Autodesk Inventor part; units mm, degrees
(part 2 of 3)
  spline S240 degree 2 poles (85.4403, 60.8078) (85.4403, 61.153) (85.7516, 61.6651) (86.3259, 61.9367) (86.6994, 61.9367) knots 0 0 0 1 2 3 3 3
  spline S241 degree 2 poles (86.6994, 61.9367) (87.087, 61.9367) (87.6557, 61.651) (87.9584, 61.1445) (87.9584, 60.8333) knots 0 0 0 1 2 3 3 3
  spline S242 degree 2 poles (87.0389, 60.8276) (87.0389, 61.2718) (86.6994, 61.2718) knots 0 0 0 1 1 1
  spline S243 degree 2 poles (86.6994, 61.2718) (86.3599, 61.2718) (86.3599, 60.8078) knots 0 0 0 1 1 1
  spline S244 degree 2 poles (86.3599, 60.8078) (86.3599, 60.3155) (86.705, 60.3155) knots 0 0 0 1 1 1
  spline S245 degree 2 poles (86.705, 60.3155) (87.0389, 60.3155) (87.0389, 60.8276) knots 0 0 0 1 1 1
  line L291 (89.7098, 59.7044) -> (89.7098, 60.8927)
  spline S246 degree 2 poles (89.7098, 60.8927) (89.7098, 61.0964) (89.5881, 61.2718) (89.4523, 61.2718) knots 0 0 0 1 2 2 2
  spline S247 degree 2 poles (89.4523, 61.2718) (89.3363, 61.2718) (89.2033, 61.0879) (89.2033, 60.9465) knots 0 0 0 1 2 2 2
  line L292 (89.2033, 60.9465) -> (89.2033, 59.7044)
  line L293 (89.2033, 59.7044) -> (88.2979, 59.7044)
  line L294 (88.2979, 59.7044) -> (88.2979, 61.883)
  line L295 (88.2979, 61.883) -> (89.2033, 61.883)
  line L296 (89.2033, 61.883) -> (89.2033, 61.5434)
  line L297 (89.2033, 61.5434) -> (89.2118, 61.5434)
  spline S248 degree 2 poles (89.2118, 61.5434) (89.3193, 61.7302) (89.6871, 61.9367) (89.9022, 61.9367) knots 0 0 0 1 2 2 2
  spline S249 degree 2 poles (89.9022, 61.9367) (90.6151, 61.9367) (90.6151, 61.0342) knots 0 0 0 1 1 1
  line L298 (90.6151, 61.0342) -> (90.6151, 59.7044)
  line L299 (90.6151, 59.7044) -> (89.7098, 59.7044)
  line L300 (91.0254, 59.7044) -> (91.0254, 61.883)
  line L301 (91.0254, 61.883) -> (91.9308, 61.883)
  line L302 (91.9308, 61.883) -> (91.9308, 59.7044)
  line L303 (91.9308, 59.7044) -> (91.0254, 59.7044)
  spline S250 degree 2 poles (91.9845, 62.4715) (91.9845, 62.2791) (91.7044, 62.0414) (91.4781, 62.0414) knots 0 0 0 1 2 2 2
  spline S251 degree 2 poles (91.4781, 62.0414) (91.2574, 62.0414) (90.9745, 62.2875) (90.9745, 62.4715) knots 0 0 0 1 2 2 2
  spline S252 degree 2 poles (90.9745, 62.4715) (90.9745, 62.6582) (91.2489, 62.8902) (91.4781, 62.8902) knots 0 0 0 1 2 2 2
  spline S253 degree 2 poles (91.4781, 62.8902) (91.7044, 62.8902) (91.9845, 62.6582) (91.9845, 62.4715) knots 0 0 0 1 2 2 2
  line L304 (93.7783, 59.7044) -> (93.7783, 60.8927)
  spline S254 degree 2 poles (93.7783, 60.8927) (93.7783, 61.0964) (93.6567, 61.2718) (93.5209, 61.2718) knots 0 0 0 1 2 2 2
  spline S255 degree 2 poles (93.5209, 61.2718) (93.4048, 61.2718) (93.2719, 61.0879) (93.2719, 60.9465) knots 0 0 0 1 2 2 2
  line L305 (93.2719, 60.9465) -> (93.2719, 59.7044)
  line L306 (93.2719, 59.7044) -> (92.3665, 59.7044)
  line L307 (92.3665, 59.7044) -> (92.3665, 61.883)
  line L308 (92.3665, 61.883) -> (93.2719, 61.883)
  line L309 (93.2719, 61.883) -> (93.2719, 61.5434)
  line L310 (93.2719, 61.5434) -> (93.2804, 61.5434)
  spline S256 degree 2 poles (93.2804, 61.5434) (93.3879, 61.7302) (93.7557, 61.9367) (93.9707, 61.9367) knots 0 0 0 1 2 2 2
  spline S257 degree 2 poles (93.9707, 61.9367) (94.6837, 61.9367) (94.6837, 61.0342) knots 0 0 0 1 1 1
  line L311 (94.6837, 61.0342) -> (94.6837, 59.7044)
  line L312 (94.6837, 59.7044) -> (93.7783, 59.7044)
  line L313 (95.0939, 59.7044) -> (95.0939, 61.883)
  line L314 (95.0939, 61.883) -> (95.9993, 61.883)
  line L315 (95.9993, 61.883) -> (95.9993, 59.7044)
  line L316 (95.9993, 59.7044) -> (95.0939, 59.7044)
  spline S258 degree 2 poles (96.0531, 62.4715) (96.0531, 62.2791) (95.773, 62.0414) (95.5466, 62.0414) knots 0 0 0 1 2 2 2
  spline S259 degree 2 poles (95.5466, 62.0414) (95.326, 62.0414) (95.043, 62.2875) (95.043, 62.4715) knots 0 0 0 1 2 2 2
  spline S260 degree 2 poles (95.043, 62.4715) (95.043, 62.6582) (95.3175, 62.8902) (95.5466, 62.8902) knots 0 0 0 1 2 2 2
  spline S261 degree 2 poles (95.5466, 62.8902) (95.773, 62.8902) (96.0531, 62.6582) (96.0531, 62.4715) knots 0 0 0 1 2 2 2
  spline S262 degree 2 poles (100.6055, 61.269) (100.6055, 60.805) (100.215, 60.092) (99.4935, 59.7044) (99.021, 59.7044) knots 0 0 0 1 2 3 3 3
  line L317 (99.021, 59.7044) -> (97.728, 59.7044)
  line L318 (97.728, 59.7044) -> (97.728, 62.7544)
  line L319 (97.728, 62.7544) -> (98.9927, 62.7544)
  spline S263 degree 2 poles (98.9927, 62.7544) (100.6055, 62.7544) (100.6055, 61.269) knots 0 0 0 1 1 1
  spline S264 degree 2 poles (99.6293, 61.2605) (99.6293, 61.4812) (99.4483, 61.8405) (99.1116, 62.0357) (98.8852, 62.0357) knots 0 0 0 1 2 3 3 3
  line L320 (98.8852, 62.0357) -> (98.6476, 62.0357)
  line L321 (98.6476, 62.0357) -> (98.6476, 60.423)
  line L322 (98.6476, 60.423) -> (98.905, 60.423)
  spline S265 degree 2 poles (98.905, 60.423) (99.2361, 60.423) (99.6293, 60.8757) (99.6293, 61.2605) knots 0 0 0 1 2 2 2
  line L323 (102.1616, 59.7044) -> (102.1616, 60.0354)
  line L324 (102.1616, 60.0354) -> (102.1531, 60.0354)
  spline S266 degree 2 poles (102.1531, 60.0354) (101.9352, 59.6506) (101.4882, 59.6506) knots 0 0 0 1 1 1
  spline S267 degree 2 poles (101.4882, 59.6506) (101.1798, 59.6506) (100.8318, 60.0156) (100.8318, 60.324) knots 0 0 0 1 2 2 2
  spline S268 degree 2 poles (100.8318, 60.324) (100.8318, 60.9663) (101.6212, 61.0681) knots 0 0 0 1 1 1
  line L325 (101.6212, 61.0681) -> (102.1616, 61.1388)
  spline S269 degree 2 poles (102.1616, 61.1388) (102.1616, 61.2464) (101.9692, 61.3822) (101.8079, 61.3822) knots 0 0 0 1 2 2 2
  spline S270 degree 2 poles (101.8079, 61.3822) (101.4429, 61.3822) (101.0355, 61.1728) knots 0 0 0 1 1 1
  line L326 (101.0355, 61.1728) -> (101.0355, 61.7613)
  spline S271 degree 2 poles (101.0355, 61.7613) (101.2109, 61.8377) (101.7457, 61.9367) (101.9352, 61.9367) knots 0 0 0 1 2 2 2
  spline S272 degree 2 poles (101.9352, 61.9367) (102.4898, 61.9367) (102.9906, 61.4614) (102.9906, 60.9068) knots 0 0 0 1 2 2 2
  line L327 (102.9906, 60.9068) -> (102.9906, 59.7044)
  line L328 (102.9906, 59.7044) -> (102.1616, 59.7044)
  spline S273 degree 2 poles (101.624, 60.4457) (101.624, 60.358) (101.7372, 60.242) (101.8419, 60.242) knots 0 0 0 1 2 2 2
  spline S274 degree 2 poles (101.8419, 60.242) (101.9833, 60.242) (102.1616, 60.4542) (102.1616, 60.6211) knots 0 0 0 1 2 2 2
  line L329 (102.1616, 60.6211) -> (102.1616, 60.7031)
  line L330 (102.1616, 60.7031) -> (101.8532, 60.6607)
  spline S275 degree 2 poles (101.8532, 60.6607) (101.624, 60.6211) (101.624, 60.4457) knots 0 0 0 1 1 1
  line L331 (104.9824, 59.7044) -> (103.9073, 59.7044)
  line L332 (103.9073, 59.7044) -> (103.1801, 61.883)
  line L333 (103.1801, 61.883) -> (104.1251, 61.883)
  line L334 (104.1251, 61.883) -> (104.3911, 60.6946)
  spline S276 degree 2 poles (104.3911, 60.6946) (104.4533, 60.4061) (104.4618, 60.2618) knots 0 0 0 1 1 1
  line L335 (104.4618, 60.2618) -> (104.4731, 60.2618)
  spline S277 degree 2 poles (104.4731, 60.2618) (104.4788, 60.3042) (104.4929, 60.3947) (104.8013, 61.883) knots 0 0 0 1 2 2 2
  line L336 (104.8013, 61.883) -> (105.7407, 61.883)
  line L337 (105.7407, 61.883) -> (104.9824, 59.7044)
  line L338 (105.9585, 59.7044) -> (105.9585, 61.883)
  line L339 (105.9585, 61.883) -> (106.8639, 61.883)
  line L340 (106.8639, 61.883) -> (106.8639, 59.7044)
  line L341 (106.8639, 59.7044) -> (105.9585, 59.7044)
  spline S278 degree 2 poles (106.9177, 62.4715) (106.9177, 62.2791) (106.6375, 62.0414) (106.4112, 62.0414) knots 0 0 0 1 2 2 2
  spline S279 degree 2 poles (106.4112, 62.0414) (106.1905, 62.0414) (105.9076, 62.2875) (105.9076, 62.4715) knots 0 0 0 1 2 2 2
  spline S280 degree 2 poles (105.9076, 62.4715) (105.9076, 62.6582) (106.182, 62.8902) (106.4112, 62.8902) knots 0 0 0 1 2 2 2
  spline S281 degree 2 poles (106.4112, 62.8902) (106.6375, 62.8902) (106.9177, 62.6582) (106.9177, 62.4715) knots 0 0 0 1 2 2 2
  line L342 (108.7539, 59.7044) -> (108.7539, 59.959)
  line L343 (108.7539, 59.959) -> (108.7454, 59.959)
  spline S282 degree 2 poles (108.7454, 59.959) (108.6379, 59.8147) (108.287, 59.6506) (108.1173, 59.6506) knots 0 0 0 1 2 2 2
  spline S283 degree 2 poles (108.1173, 59.6506) (107.84, 59.6506) (107.4128, 59.9251) (107.2034, 60.4202) (107.2034, 60.7541) knots 0 0 0 1 2 3 3 3
  spline S284 degree 2 poles (107.2034, 60.7541) (107.2034, 61.1021) (107.4552, 61.6396) (107.9107, 61.9367) (108.1937, 61.9367) knots 0 0 0 1 2 3 3 3
  spline S285 degree 2 poles (108.1937, 61.9367) (108.3266, 61.9367) (108.553, 61.8603) (108.7228, 61.7302) (108.7454, 61.6651) knots 0 0 0 1 2 3 3 3
  line L344 (108.7454, 61.6651) -> (108.7539, 61.6651)
  line L345 (108.7539, 61.6651) -> (108.7539, 62.9298)
  line L346 (108.7539, 62.9298) -> (109.6593, 62.9298)
  line L347 (109.6593, 62.9298) -> (109.6593, 59.7044)
  line L348 (109.6593, 59.7044) -> (108.7539, 59.7044)
  spline S286 degree 2 poles (108.7737, 60.8587) (108.7737, 61.054) (108.6011, 61.2718) (108.454, 61.2718) knots 0 0 0 1 2 2 2
  spline S287 degree 2 poles (108.454, 61.2718) (108.3068, 61.2718) (108.1229, 61.003) (108.1229, 60.7767) knots 0 0 0 1 2 2 2
  spline S288 degree 2 poles (108.1229, 60.7767) (108.1229, 60.3155) (108.4427, 60.3155) knots 0 0 0 1 1 1
  spline S289 degree 2 poles (108.4427, 60.3155) (108.5926, 60.3155) (108.7737, 60.5645) (108.7737, 60.8022) knots 0 0 0 1 2 2 2
  line L349 (108.7737, 60.8022) -> (108.7737, 60.8587)
  spline S290 degree 2 poles (110.8787, 60.5362) (110.9013, 60.3947) (111.1786, 60.2363) (111.4049, 60.2363) knots 0 0 0 1 2 2 2
  spline S291 degree 2 poles (111.4049, 60.2363) (111.7218, 60.2363) (112.0048, 60.358) knots 0 0 0 1 1 1
  line L350 (112.0048, 60.358) -> (112.0048, 59.7836)
  spline S292 degree 2 poles (112.0048, 59.7836) (111.6766, 59.6506) (111.2041, 59.6506) knots 0 0 0 1 1 1
  spline S293 degree 2 poles (111.2041, 59.6506) (110.6354, 59.6506) (110.0016, 60.2335) (110.0016, 60.7456) knots 0 0 0 1 2 2 2
  spline S294 degree 2 poles (110.0016, 60.7456) (110.0016, 61.0964) (110.2789, 61.6311) (110.8249, 61.9367) (111.156, 61.9367) knots 0 0 0 1 2 3 3 3
  spline S295 degree 2 poles (111.156, 61.9367) (111.4927, 61.9367) (111.9736, 61.6736) (112.2226, 61.1954) (112.2226, 60.8757) knots 0 0 0 1 2 3 3 3
  line L351 (112.2226, 60.8757) -> (112.2226, 60.5362)
  line L352 (112.2226, 60.5362) -> (110.8787, 60.5362)
  spline S296 degree 2 poles (111.4219, 61.0115) (111.4219, 61.3878) (111.1531, 61.3878) knots 0 0 0 1 1 1
  spline S297 degree 2 poles (111.1531, 61.3878) (111.04, 61.3878) (110.8872, 61.1813) (110.873, 61.0115) knots 0 0 0 1 2 2 2
  line L353 (110.873, 61.0115) -> (111.4219, 61.0115)
  spline S298 degree 2 poles (69.93, 54.8061) (69.93, 54.642) (69.7603, 54.3506) (69.4689, 54.1836) (69.3076, 54.1836) knots 0 0 0 1 2 3 3 3
  spline S299 degree 2 poles (69.3076, 54.1836) (69.0558, 54.1836) (68.6936, 54.5458) (68.6936, 54.8061) knots 0 0 0 1 2 2 2
  spline S300 degree 2 poles (68.6936, 54.8061) (68.6936, 55.0579) (69.0501, 55.42) (69.3076, 55.42) knots 0 0 0 1 2 2 2
  spline S301 degree 2 poles (69.3076, 55.42) (69.5707, 55.42) (69.93, 55.0522) (69.93, 54.8061) knots 0 0 0 1 2 2 2
  spline S302 degree 2 poles (80.076, 53.8498) (79.6968, 53.714) (79.2017, 53.714) knots 0 0 0 1 1 1
  spline S303 degree 2 poles (79.2017, 53.714) (78.7151, 53.714) (78.0106, 54.0874) (77.6371, 54.7721) (77.6371, 55.222) knots 0 0 0 1 2 3 3 3
  spline S304 degree 2 poles (77.6371, 55.222) (77.6371, 55.7058) (78.053, 56.4584) (78.8141, 56.8686) (79.3092, 56.8686) knots 0 0 0 1 2 3 3 3
  spline S305 degree 2 poles (79.3092, 56.8686) (79.7053, 56.8686) (80.076, 56.7725) knots 0 0 0 1 1 1
  line L354 (80.076, 56.7725) -> (80.076, 55.9237)
  spline S306 degree 2 poles (80.076, 55.9237) (79.9486, 56) (79.595, 56.0849) (79.4167, 56.0849) knots 0 0 0 1 2 2 2
  spline S307 degree 2 poles (79.4167, 56.0849) (79.0404, 56.0849) (78.6104, 55.6549) (78.6104, 55.2871) knots 0 0 0 1 2 2 2
  spline S308 degree 2 poles (78.6104, 55.2871) (78.6104, 54.9221) (79.0404, 54.4977) (79.4026, 54.4977) knots 0 0 0 1 2 2 2
  spline S309 degree 2 poles (79.4026, 54.4977) (79.7364, 54.4977) (80.076, 54.6703) knots 0 0 0 1 1 1
  line L355 (80.076, 54.6703) -> (80.076, 53.8498)
  spline S310 degree 2 poles (82.8911, 54.8966) (82.8911, 54.3449) (82.2262, 53.714) (81.6292, 53.714) knots 0 0 0 1 2 2 2
  spline S311 degree 2 poles (81.6292, 53.714) (81.0351, 53.714) (80.373, 54.3279) (80.373, 54.8712) knots 0 0 0 1 2 2 2
  spline S312 degree 2 poles (80.373, 54.8712) (80.373, 55.2163) (80.6843, 55.7284) (81.2586, 56) (81.6321, 56) knots 0 0 0 1 2 3 3 3
  spline S313 degree 2 poles (81.6321, 56) (82.0197, 56) (82.5884, 55.7143) (82.8911, 55.2078) (82.8911, 54.8966) knots 0 0 0 1 2 3 3 3
  spline S314 degree 2 poles (81.9716, 54.891) (81.9716, 55.3352) (81.6321, 55.3352) knots 0 0 0 1 1 1
  spline S315 degree 2 poles (81.6321, 55.3352) (81.2926, 55.3352) (81.2926, 54.8712) knots 0 0 0 1 1 1
  spline S316 degree 2 poles (81.2926, 54.8712) (81.2926, 54.3789) (81.6377, 54.3789) knots 0 0 0 1 1 1
  spline S317 degree 2 poles (81.6377, 54.3789) (81.9716, 54.3789) (81.9716, 54.891) knots 0 0 0 1 1 1
  spline S318 degree 2 poles (85.0018, 54.492) (85.0018, 54.1214) (84.4359, 53.714) (83.9323, 53.714) knots 0 0 0 1 2 2 2
  spline S319 degree 2 poles (83.9323, 53.714) (83.7852, 53.714) (83.3523, 53.7734) (83.2165, 53.8158) knots 0 0 0 1 2 2 2
  line L356 (83.2165, 53.8158) -> (83.2165, 54.4524)
  spline S320 degree 2 poles (83.2165, 54.4524) (83.6183, 54.2742) (83.8899, 54.2742) knots 0 0 0 1 1 1
  spline S321 degree 2 poles (83.8899, 54.2742) (84.1558, 54.2742) (84.1558, 54.4128) knots 0 0 0 1 1 1
  spline S322 degree 2 poles (84.1558, 54.4128) (84.1558, 54.4694) (84.0313, 54.5458) (83.771, 54.6307) knots 0 0 0 1 2 2 2
  spline S323 degree 2 poles (83.771, 54.6307) (83.4796, 54.724) (83.2165, 55.0268) (83.2165, 55.2673) knots 0 0 0 1 2 2 2
  spline S324 degree 2 poles (83.2165, 55.2673) (83.2165, 55.6068) (83.7569, 56) (84.2435, 56) knots 0 0 0 1 2 2 2
  spline S325 degree 2 poles (84.2435, 56) (84.5293, 56) (84.849, 55.918) knots 0 0 0 1 1 1
  line L357 (84.849, 55.918) -> (84.849, 55.3069)
  spline S326 degree 2 poles (84.849, 55.3069) (84.7132, 55.3635) (84.3935, 55.4398) (84.286, 55.4398) knots 0 0 0 1 2 2 2
  spline S327 degree 2 poles (84.286, 55.4398) (84.1954, 55.4398) (84.0879, 55.3804) (84.0879, 55.3267) knots 0 0 0 1 2 2 2
  spline S328 degree 2 poles (84.0879, 55.3267) (84.0879, 55.2644) (84.2039, 55.188) (84.3765, 55.1343) knots 0 0 0 1 2 2 2
  spline S329 degree 2 poles (84.3765, 55.1343) (84.7104, 55.0381) (85.0018, 54.7325) (85.0018, 54.492) knots 0 0 0 1 2 2 2
  spline S330 degree 2 poles (86.1165, 54.5995) (86.1392, 54.4581) (86.4164, 54.2996) (86.6428, 54.2996) knots 0 0 0 1 2 2 2
  spline S331 degree 2 poles (86.6428, 54.2996) (86.9597, 54.2996) (87.2426, 54.4213) knots 0 0 0 1 1 1
  line L358 (87.2426, 54.4213) -> (87.2426, 53.8469)
  spline S332 degree 2 poles (87.2426, 53.8469) (86.9144, 53.714) (86.4419, 53.714) knots 0 0 0 1 1 1
  spline S333 degree 2 poles (86.4419, 53.714) (85.8732, 53.714) (85.2394, 54.2968) (85.2394, 54.8089) knots 0 0 0 1 2 2 2
  spline S334 degree 2 poles (85.2394, 54.8089) (85.2394, 55.1597) (85.5167, 55.6945) (86.0628, 56) (86.3938, 56) knots 0 0 0 1 2 3 3 3
  spline S335 degree 2 poles (86.3938, 56) (86.7305, 56) (87.2115, 55.7369) (87.4605, 55.2588) (87.4605, 54.9391) knots 0 0 0 1 2 3 3 3
  line L359 (87.4605, 54.9391) -> (87.4605, 54.5995)
  line L360 (87.4605, 54.5995) -> (86.1165, 54.5995)
  spline S336 degree 2 poles (86.6598, 55.0749) (86.6598, 55.4512) (86.391, 55.4512) knots 0 0 0 1 1 1
  spline S337 degree 2 poles (86.391, 55.4512) (86.2778, 55.4512) (86.125, 55.2446) (86.1109, 55.0749) knots 0 0 0 1 2 2 2
  line L361 (86.1109, 55.0749) -> (86.6598, 55.0749)
  line L362 (89.1863, 53.7677) -> (89.1863, 54.956)
  spline S338 degree 2 poles (89.1863, 54.956) (89.1863, 55.1597) (89.0647, 55.3352) (88.9289, 55.3352) knots 0 0 0 1 2 2 2
  spline S339 degree 2 poles (88.9289, 55.3352) (88.8129, 55.3352) (88.6799, 55.1513) (88.6799, 55.0098) knots 0 0 0 1 2 2 2
  line L363 (88.6799, 55.0098) -> (88.6799, 53.7677)
  line L364 (88.6799, 53.7677) -> (87.7745, 53.7677)
  line L365 (87.7745, 53.7677) -> (87.7745, 55.9463)
  line L366 (87.7745, 55.9463) -> (88.6799, 55.9463)
  line L367 (88.6799, 55.9463) -> (88.6799, 55.6068)
  line L368 (88.6799, 55.6068) -> (88.6884, 55.6068)
  spline S340 degree 2 poles (88.6884, 55.6068) (88.7959, 55.7935) (89.1637, 56) (89.3787, 56) knots 0 0 0 1 2 2 2
  spline S341 degree 2 poles (89.3787, 56) (90.0917, 56) (90.0917, 55.0975) knots 0 0 0 1 1 1
  line L369 (90.0917, 55.0975) -> (90.0917, 53.7677)
  line L370 (90.0917, 53.7677) -> (89.1863, 53.7677)
  spline S342 degree 2 poles (92.0355, 53.796) (91.9732, 53.7677) (91.6931, 53.714) (91.4951, 53.714) knots 0 0 0 1 2 2 2
  spline S343 degree 2 poles (91.4951, 53.714) (91.1159, 53.714) (90.6887, 54.1299) (90.6887, 54.5175) knots 0 0 0 1 2 2 2
  line L371 (90.6887, 54.5175) -> (90.6887, 55.3182)
  line L372 (90.6887, 55.3182) -> (90.3464, 55.3182)
  line L373 (90.3464, 55.3182) -> (90.3464, 55.9463)
  line L374 (90.3464, 55.9463) -> (90.6887, 55.9463)
  line L375 (90.6887, 55.9463) -> (90.6887, 56.3735)
  line L376 (90.6887, 56.3735) -> (91.5828, 56.6197)
  line L377 (91.5828, 56.6197) -> (91.5828, 55.9463)
  line L378 (91.5828, 55.9463) -> (92.0355, 55.9463)
  line L379 (92.0355, 55.9463) -> (92.0355, 55.3182)
  line L380 (92.0355, 55.3182) -> (91.5828, 55.3182)
  line L381 (91.5828, 55.3182) -> (91.5828, 54.6646)
  spline S344 degree 2 poles (91.5828, 54.6646) (91.5828, 54.3789) (91.8091, 54.3789) knots 0 0 0 1 1 1
  spline S345 degree 2 poles (91.8091, 54.3789) (91.9166, 54.3789) (92.0355, 54.4241) knots 0 0 0 1 1 1
  line L382 (92.0355, 54.4241) -> (92.0355, 53.796)
  line L383 (92.3184, 53.7677) -> (92.3184, 55.9463)
  line L384 (92.3184, 55.9463) -> (93.2238, 55.9463)
  line L385 (93.2238, 55.9463) -> (93.2238, 53.7677)
  line L386 (93.2238, 53.7677) -> (92.3184, 53.7677)
  spline S346 degree 2 poles (93.2775, 56.5348) (93.2775, 56.3424) (92.9974, 56.1047) (92.7711, 56.1047) knots 0 0 0 1 2 2 2
  spline S347 degree 2 poles (92.7711, 56.1047) (92.5504, 56.1047) (92.2675, 56.3509) (92.2675, 56.5348) knots 0 0 0 1 2 2 2
  spline S348 degree 2 poles (92.2675, 56.5348) (92.2675, 56.7215) (92.5419, 56.9535) (92.7711, 56.9535) knots 0 0 0 1 2 2 2
  spline S349 degree 2 poles (92.7711, 56.9535) (92.9974, 56.9535) (93.2775, 56.7215) (93.2775, 56.5348) knots 0 0 0 1 2 2 2
  line L387 (95.0713, 53.7677) -> (95.0713, 54.956)
  spline S350 degree 2 poles (95.0713, 54.956) (95.0713, 55.1597) (94.9497, 55.3352) (94.8138, 55.3352) knots 0 0 0 1 2 2 2
  spline S351 degree 2 poles (94.8138, 55.3352) (94.6978, 55.3352) (94.5649, 55.1513) (94.5649, 55.0098) knots 0 0 0 1 2 2 2
  line L388 (94.5649, 55.0098) -> (94.5649, 53.7677)
  line L389 (94.5649, 53.7677) -> (93.6595, 53.7677)
  line L390 (93.6595, 53.7677) -> (93.6595, 55.9463)
  line L391 (93.6595, 55.9463) -> (94.5649, 55.9463)
  line L392 (94.5649, 55.9463) -> (94.5649, 55.6068)
  line L393 (94.5649, 55.6068) -> (94.5734, 55.6068)
  spline S352 degree 2 poles (94.5734, 55.6068) (94.6809, 55.7935) (95.0487, 56) (95.2637, 56) knots 0 0 0 1 2 2 2
  spline S353 degree 2 poles (95.2637, 56) (95.9767, 56) (95.9767, 55.0975) knots 0 0 0 1 1 1
  line L394 (95.9767, 55.0975) -> (95.9767, 53.7677)
  line L395 (95.9767, 53.7677) -> (95.0713, 53.7677)
  line L396 (96.3869, 53.7677) -> (96.3869, 55.9463)
  line L397 (96.3869, 55.9463) -> (97.2923, 55.9463)
  line L398 (97.2923, 55.9463) -> (97.2923, 53.7677)
  line L399 (97.2923, 53.7677) -> (96.3869, 53.7677)
  spline S354 degree 2 poles (97.3461, 56.5348) (97.3461, 56.3424) (97.066, 56.1047) (96.8396, 56.1047) knots 0 0 0 1 2 2 2
  spline S355 degree 2 poles (96.8396, 56.1047) (96.6189, 56.1047) (96.336, 56.3509) (96.336, 56.5348) knots 0 0 0 1 2 2 2
  spline S356 degree 2 poles (96.336, 56.5348) (96.336, 56.7215) (96.6105, 56.9535) (96.8396, 56.9535) knots 0 0 0 1 2 2 2
  spline S357 degree 2 poles (96.8396, 56.9535) (97.066, 56.9535) (97.3461, 56.7215) (97.3461, 56.5348) knots 0 0 0 1 2 2 2
  line L400 (100.9337, 53.7677) -> (100.8007, 54.3279)
  line L401 (100.8007, 54.3279) -> (99.8896, 54.3279)
  line L402 (99.8896, 54.3279) -> (99.7453, 53.7677)
  line L403 (99.7453, 53.7677) -> (98.7523, 53.7677)
  line L404 (98.7523, 53.7677) -> (99.8019, 56.8177)
  line L405 (99.8019, 56.8177) -> (100.9421, 56.8177)
  line L406 (100.9421, 56.8177) -> (101.9324, 53.7677)
  line L407 (101.9324, 53.7677) -> (100.9337, 53.7677)
  line L408 (100.3565, 56.1528) -> (100.3367, 56.1528)
  spline S358 degree 2 poles (100.3367, 56.1528) (100.331, 56.1019) (100.2801, 55.8671) (100.0481, 54.9815) knots 0 0 0 1 2 2 2
  line L409 (100.0481, 54.9815) -> (100.6309, 54.9815)
  line L410 (100.6309, 54.9815) -> (100.4187, 55.8105)
  spline S359 degree 2 poles (100.4187, 55.8105) (100.3734, 55.9944) (100.3565, 56.1528) knots 0 0 0 1 1 1
  line L411 (102.2068, 53.7677) -> (102.2068, 56.9931)
  line L412 (102.2068, 56.9931) -> (103.1122, 56.9931)
  line L413 (103.1122, 56.9931) -> (103.1122, 53.7677)
  line L414 (103.1122, 53.7677) -> (102.2068, 53.7677)
  spline S360 degree 2 poles (104.3288, 54.5995) (104.3515, 54.4581) (104.6287, 54.2996) (104.8551, 54.2996) knots 0 0 0 1 2 2 2
  spline S361 degree 2 poles (104.8551, 54.2996) (105.172, 54.2996) (105.4549, 54.4213) knots 0 0 0 1 1 1
  line L415 (105.4549, 54.4213) -> (105.4549, 53.8469)
  spline S362 degree 2 poles (105.4549, 53.8469) (105.1267, 53.714) (104.6542, 53.714) knots 0 0 0 1 1 1
  spline S363 degree 2 poles (104.6542, 53.714) (104.0855, 53.714) (103.4517, 54.2968) (103.4517, 54.8089) knots 0 0 0 1 2 2 2
  spline S364 degree 2 poles (103.4517, 54.8089) (103.4517, 55.1597) (103.729, 55.6945) (104.2751, 56) (104.6061, 56) knots 0 0 0 1 2 3 3 3
  spline S365 degree 2 poles (104.6061, 56) (104.9428, 56) (105.4238, 55.7369) (105.6728, 55.2588) (105.6728, 54.9391) knots 0 0 0 1 2 3 3 3
  line L416 (105.6728, 54.9391) -> (105.6728, 54.5995)
  line L417 (105.6728, 54.5995) -> (104.3288, 54.5995)
  spline S366 degree 2 poles (104.8721, 55.0749) (104.8721, 55.4512) (104.6033, 55.4512) knots 0 0 0 1 1 1
  spline S367 degree 2 poles (104.6033, 55.4512) (104.4901, 55.4512) (104.3373, 55.2446) (104.3232, 55.0749) knots 0 0 0 1 2 2 2
  line L418 (104.3232, 55.0749) -> (104.8721, 55.0749)
  spline S368 degree 2 poles (107.758, 54.492) (107.758, 54.1214) (107.1921, 53.714) (106.6885, 53.714) knots 0 0 0 1 2 2 2
  spline S369 degree 2 poles (106.6885, 53.714) (106.5414, 53.714) (106.1085, 53.7734) (105.9727, 53.8158) knots 0 0 0 1 2 2 2
  line L419 (105.9727, 53.8158) -> (105.9727, 54.4524)
  spline S370 degree 2 poles (105.9727, 54.4524) (106.3744, 54.2742) (106.646, 54.2742) knots 0 0 0 1 1 1
  spline S371 degree 2 poles (106.646, 54.2742) (106.912, 54.2742) (106.912, 54.4128) knots 0 0 0 1 1 1
  spline S372 degree 2 poles (106.912, 54.4128) (106.912, 54.4694) (106.7875, 54.5458) (106.5272, 54.6307) knots 0 0 0 1 2 2 2
  spline S373 degree 2 poles (106.5272, 54.6307) (106.2358, 54.724) (105.9727, 55.0268) (105.9727, 55.2673) knots 0 0 0 1 2 2 2
  spline S374 degree 2 poles (105.9727, 55.2673) (105.9727, 55.6068) (106.5131, 56) (106.9997, 56) knots 0 0 0 1 2 2 2
  spline S375 degree 2 poles (106.9997, 56) (107.2855, 56) (107.6052, 55.918) knots 0 0 0 1 1 1
  line L420 (107.6052, 55.918) -> (107.6052, 55.3069)
  spline S376 degree 2 poles (107.6052, 55.3069) (107.4694, 55.3635) (107.1497, 55.4398) (107.0421, 55.4398) knots 0 0 0 1 2 2 2
  spline S377 degree 2 poles (107.0421, 55.4398) (106.9516, 55.4398) (106.8441, 55.3804) (106.8441, 55.3267) knots 0 0 0 1 2 2 2
  spline S378 degree 2 poles (106.8441, 55.3267) (106.8441, 55.2644) (106.9601, 55.188) (107.1327, 55.1343) knots 0 0 0 1 2 2 2
  spline S379 degree 2 poles (107.1327, 55.1343) (107.4665, 55.0381) (107.758, 54.7325) (107.758, 54.492) knots 0 0 0 1 2 2 2
  spline S380 degree 2 poles (109.863, 54.492) (109.863, 54.1214) (109.2971, 53.714) (108.7935, 53.714) knots 0 0 0 1 2 2 2
  spline S381 degree 2 poles (108.7935, 53.714) (108.6464, 53.714) (108.2135, 53.7734) (108.0777, 53.8158) knots 0 0 0 1 2 2 2
  line L421 (108.0777, 53.8158) -> (108.0777, 54.4524)
  spline S382 degree 2 poles (108.0777, 54.4524) (108.4794, 54.2742) (108.751, 54.2742) knots 0 0 0 1 1 1
  spline S383 degree 2 poles (108.751, 54.2742) (109.017, 54.2742) (109.017, 54.4128) knots 0 0 0 1 1 1
  spline S384 degree 2 poles (109.017, 54.4128) (109.017, 54.4694) (108.8925, 54.5458) (108.6322, 54.6307) knots 0 0 0 1 2 2 2
  spline S385 degree 2 poles (108.6322, 54.6307) (108.3408, 54.724) (108.0777, 55.0268) (108.0777, 55.2673) knots 0 0 0 1 2 2 2
  spline S386 degree 2 poles (108.0777, 55.2673) (108.0777, 55.6068) (108.6181, 56) (109.1047, 56) knots 0 0 0 1 2 2 2
  spline S387 degree 2 poles (109.1047, 56) (109.3905, 56) (109.7102, 55.918) knots 0 0 0 1 1 1
  line L422 (109.7102, 55.918) -> (109.7102, 55.3069)
  spline S388 degree 2 poles (109.7102, 55.3069) (109.5744, 55.3635) (109.2547, 55.4398) (109.1471, 55.4398) knots 0 0 0 1 2 2 2
  spline S389 degree 2 poles (109.1471, 55.4398) (109.0566, 55.4398) (108.9491, 55.3804) (108.9491, 55.3267) knots 0 0 0 1 2 2 2
  spline S390 degree 2 poles (108.9491, 55.3267) (108.9491, 55.2644) (109.0651, 55.188) (109.2377, 55.1343) knots 0 0 0 1 2 2 2
  spline S391 degree 2 poles (109.2377, 55.1343) (109.5715, 55.0381) (109.863, 54.7325) (109.863, 54.492) knots 0 0 0 1 2 2 2
  line L423 (111.4049, 53.7677) -> (111.4049, 54.0987)
  line L424 (111.4049, 54.0987) -> (111.3965, 54.0987)
  spline S392 degree 2 poles (111.3965, 54.0987) (111.1786, 53.714) (110.7316, 53.714) knots 0 0 0 1 1 1
  spline S393 degree 2 poles (110.7316, 53.714) (110.4232, 53.714) (110.0752, 54.0789) (110.0752, 54.3873) knots 0 0 0 1 2 2 2
  spline S394 degree 2 poles (110.0752, 54.3873) (110.0752, 55.0296) (110.8645, 55.1314) knots 0 0 0 1 1 1
  line L425 (110.8645, 55.1314) -> (111.4049, 55.2022)
  spline S395 degree 2 poles (111.4049, 55.2022) (111.4049, 55.3097) (111.2125, 55.4455) (111.0513, 55.4455) knots 0 0 0 1 2 2 2
  spline S396 degree 2 poles (111.0513, 55.4455) (110.6863, 55.4455) (110.2789, 55.2361) knots 0 0 0 1 1 1
  line L426 (110.2789, 55.2361) -> (110.2789, 55.8246)
  spline S397 degree 2 poles (110.2789, 55.8246) (110.4543, 55.901) (110.989, 56) (111.1786, 56) knots 0 0 0 1 2 2 2
  spline S398 degree 2 poles (111.1786, 56) (111.7331, 56) (112.2339, 55.5247) (112.2339, 54.9702) knots 0 0 0 1 2 2 2
  line L427 (112.2339, 54.9702) -> (112.2339, 53.7677)
  line L428 (112.2339, 53.7677) -> (111.4049, 53.7677)
  spline S399 degree 2 poles (110.8674, 54.509) (110.8674, 54.4213) (110.9805, 54.3053) (111.0852, 54.3053) knots 0 0 0 1 2 2 2
  spline S400 degree 2 poles (111.0852, 54.3053) (111.2267, 54.3053) (111.4049, 54.5175) (111.4049, 54.6844) knots 0 0 0 1 2 2 2
  line L429 (111.4049, 54.6844) -> (111.4049, 54.7665)
  line L430 (111.4049, 54.7665) -> (111.0965, 54.724)
  spline S401 degree 2 poles (111.0965, 54.724) (110.8674, 54.6844) (110.8674, 54.509) knots 0 0 0 1 1 1
  line L431 (114.0532, 53.7677) -> (114.0532, 54.956)
  spline S402 degree 2 poles (114.0532, 54.956) (114.0532, 55.1597) (113.9315, 55.3352) (113.7957, 55.3352) knots 0 0 0 1 2 2 2
  spline S403 degree 2 poles (113.7957, 55.3352) (113.6797, 55.3352) (113.5467, 55.1513) (113.5467, 55.0098) knots 0 0 0 1 2 2 2
  line L432 (113.5467, 55.0098) -> (113.5467, 53.7677)
  line L433 (113.5467, 53.7677) -> (112.6414, 53.7677)
  line L434 (112.6414, 53.7677) -> (112.6414, 55.9463)
  line L435 (112.6414, 55.9463) -> (113.5467, 55.9463)
  line L436 (113.5467, 55.9463) -> (113.5467, 55.6068)
  line L437 (113.5467, 55.6068) -> (113.5552, 55.6068)
  spline S404 degree 2 poles (113.5552, 55.6068) (113.6627, 55.7935) (114.0305, 56) (114.2456, 56) knots 0 0 0 1 2 2 2
  spline S405 degree 2 poles (114.2456, 56) (114.9586, 56) (114.9586, 55.0975) knots 0 0 0 1 1 1
  line L438 (114.9586, 55.0975) -> (114.9586, 53.7677)
  line L439 (114.9586, 53.7677) -> (114.0532, 53.7677)
  line L440 (116.8231, 53.7677) -> (116.8231, 54.0224)
  line L441 (116.8231, 54.0224) -> (116.8146, 54.0224)
  spline S406 degree 2 poles (116.8146, 54.0224) (116.7071, 53.8781) (116.3562, 53.714) (116.1865, 53.714) knots 0 0 0 1 2 2 2
  spline S407 degree 2 poles (116.1865, 53.714) (115.9092, 53.714) (115.482, 53.9884) (115.2726, 54.4835) (115.2726, 54.8174) knots 0 0 0 1 2 3 3 3
  spline S408 degree 2 poles (115.2726, 54.8174) (115.2726, 55.1654) (115.5244, 55.703) (115.9799, 56) (116.2629, 56) knots 0 0 0 1 2 3 3 3
  spline S409 degree 2 poles (116.2629, 56) (116.3959, 56) (116.6222, 55.9237) (116.792, 55.7935) (116.8146, 55.7284) knots 0 0 0 1 2 3 3 3
  line L442 (116.8146, 55.7284) -> (116.8231, 55.7284)
  line L443 (116.8231, 55.7284) -> (116.8231, 56.9931)
  line L444 (116.8231, 56.9931) -> (117.7285, 56.9931)
  line L445 (117.7285, 56.9931) -> (117.7285, 53.7677)
  line L446 (117.7285, 53.7677) -> (116.8231, 53.7677)
  spline S410 degree 2 poles (116.8429, 54.9221) (116.8429, 55.1173) (116.6703, 55.3352) (116.5232, 55.3352) knots 0 0 0 1 2 2 2
  spline S411 degree 2 poles (116.5232, 55.3352) (116.376, 55.3352) (116.1921, 55.0664) (116.1921, 54.84) knots 0 0 0 1 2 2 2
  spline S412 degree 2 poles (116.1921, 54.84) (116.1921, 54.3789) (116.5119, 54.3789) knots 0 0 0 1 1 1
  spline S413 degree 2 poles (116.5119, 54.3789) (116.6618, 54.3789) (116.8429, 54.6278) (116.8429, 54.8655) knots 0 0 0 1 2 2 2
  line L447 (116.8429, 54.8655) -> (116.8429, 54.9221)
  spline S414 degree 2 poles (119.8052, 55.1711) (119.7542, 55.1937) (119.5788, 55.2305) (119.5222, 55.2305) knots 0 0 0 1 2 2 2
  spline S415 degree 2 poles (119.5222, 55.2305) (119.0724, 55.2305) (119.0724, 54.7127) knots 0 0 0 1 1 1
  line L448 (119.0724, 54.7127) -> (119.0724, 53.7677)
  line L449 (119.0724, 53.7677) -> (118.167, 53.7677)
  line L450 (118.167, 53.7677) -> (118.167, 55.9463)
  line L451 (118.167, 55.9463) -> (119.0724, 55.9463)
  line L452 (119.0724, 55.9463) -> (119.0724, 55.5643)
  line L453 (119.0724, 55.5643) -> (119.0809, 55.5643)
  spline S416 degree 2 poles (119.0809, 55.5643) (119.1629, 55.7709) (119.4713, 55.9859) (119.675, 55.9859) knots 0 0 0 1 2 2 2
  spline S417 degree 2 poles (119.675, 55.9859) (119.7486, 55.9859) (119.8052, 55.9604) knots 0 0 0 1 1 1
  line L454 (119.8052, 55.9604) -> (119.8052, 55.1711)
  spline S418 degree 2 poles (122.4874, 54.8966) (122.4874, 54.3449) (121.8225, 53.714) (121.2255, 53.714) knots 0 0 0 1 2 2 2
  spline S419 degree 2 poles (121.2255, 53.714) (120.6313, 53.714) (119.9693, 54.3279) (119.9693, 54.8712) knots 0 0 0 1 2 2 2
  spline S420 degree 2 poles (119.9693, 54.8712) (119.9693, 55.2163) (120.2805, 55.7284) (120.8548, 56) (121.2283, 56) knots 0 0 0 1 2 3 3 3
  spline S421 degree 2 poles (121.2283, 56) (121.6159, 56) (122.1846, 55.7143) (122.4874, 55.2078) (122.4874, 54.8966) knots 0 0 0 1 2 3 3 3
  spline S422 degree 2 poles (121.5678, 54.891) (121.5678, 55.3352) (121.2283, 55.3352) knots 0 0 0 1 1 1
  spline S423 degree 2 poles (121.2283, 55.3352) (120.8888, 55.3352) (120.8888, 54.8712) knots 0 0 0 1 1 1
  spline S424 degree 2 poles (120.8888, 54.8712) (120.8888, 54.3789) (121.234, 54.3789) knots 0 0 0 1 1 1
  spline S425 degree 2 poles (121.234, 54.3789) (121.5678, 54.3789) (121.5678, 54.891) knots 0 0 0 1 1 1
  spline S426 degree 2 poles (69.93, 48.8694) (69.93, 48.7053) (69.7603, 48.4139) (69.4689, 48.247) (69.3076, 48.247) knots 0 0 0 1 2 3 3 3
  spline S427 degree 2 poles (69.3076, 48.247) (69.0558, 48.247) (68.6936, 48.6091) (68.6936, 48.8694) knots 0 0 0 1 2 2 2
  spline S428 degree 2 poles (68.6936, 48.8694) (68.6936, 49.1212) (69.0501, 49.4834) (69.3076, 49.4834) knots 0 0 0 1 2 2 2
  spline S429 degree 2 poles (69.3076, 49.4834) (69.5707, 49.4834) (69.93, 49.1156) (69.93, 48.8694) knots 0 0 0 1 2 2 2
  spline S430 degree 2 poles (80.6843, 49.3957) (80.6843, 48.9317) (80.2938, 48.2187) (79.5723, 47.8311) (79.0998, 47.8311) knots 0 0 0 1 2 3 3 3
  line L455 (79.0998, 47.8311) -> (77.8068, 47.8311)
  line L456 (77.8068, 47.8311) -> (77.8068, 50.8811)
  line L457 (77.8068, 50.8811) -> (79.0715, 50.8811)
  spline S431 degree 2 poles (79.0715, 50.8811) (80.6843, 50.8811) (80.6843, 49.3957) knots 0 0 0 1 1 1
  spline S432 degree 2 poles (79.7081, 49.3872) (79.7081, 49.6079) (79.5271, 49.9672) (79.1904, 50.1624) (78.964, 50.1624) knots 0 0 0 1 2 3 3 3
  line L458 (78.964, 50.1624) -> (78.7264, 50.1624)
  line L459 (78.7264, 50.1624) -> (78.7264, 48.5497)
  line L460 (78.7264, 48.5497) -> (78.9838, 48.5497)
  spline S433 degree 2 poles (78.9838, 48.5497) (79.3149, 48.5497) (79.7081, 49.0024) (79.7081, 49.3872) knots 0 0 0 1 2 2 2
  spline S434 degree 2 poles (81.8132, 48.6629) (81.8358, 48.5214) (82.1131, 48.363) (82.3394, 48.363) knots 0 0 0 1 2 2 2
  spline S435 degree 2 poles (82.3394, 48.363) (82.6563, 48.363) (82.9392, 48.4846) knots 0 0 0 1 1 1
  line L461 (82.9392, 48.4846) -> (82.9392, 47.9103)
  spline S436 degree 2 poles (82.9392, 47.9103) (82.611, 47.7773) (82.1385, 47.7773) knots 0 0 0 1 1 1
  spline S437 degree 2 poles (82.1385, 47.7773) (81.5698, 47.7773) (80.9361, 48.3601) (80.9361, 48.8722) knots 0 0 0 1 2 2 2
  spline S438 degree 2 poles (80.9361, 48.8722) (80.9361, 49.2231) (81.2133, 49.7578) (81.7594, 50.0634) (82.0904, 50.0634) knots 0 0 0 1 2 3 3 3
  spline S439 degree 2 poles (82.0904, 50.0634) (82.4271, 50.0634) (82.9081, 49.8003) (83.1571, 49.3221) (83.1571, 49.0024) knots 0 0 0 1 2 3 3 3
  line L462 (83.1571, 49.0024) -> (83.1571, 48.6629)
  line L463 (83.1571, 48.6629) -> (81.8132, 48.6629)
  spline S440 degree 2 poles (82.3564, 49.1382) (82.3564, 49.5145) (82.0876, 49.5145) knots 0 0 0 1 1 1
  spline S441 degree 2 poles (82.0876, 49.5145) (81.9744, 49.5145) (81.8216, 49.308) (81.8075, 49.1382) knots 0 0 0 1 2 2 2
  line L464 (81.8075, 49.1382) -> (82.3564, 49.1382)
  line L465 (83.4711, 47.8311) -> (83.4711, 51.0565)
  line L466 (83.4711, 51.0565) -> (84.3765, 51.0565)
  line L467 (84.3765, 51.0565) -> (84.3765, 47.8311)
  line L468 (84.3765, 47.8311) -> (83.4711, 47.8311)
  spline S442 degree 2 poles (88.6007, 49.8766) (88.6007, 49.5626) (88.2838, 49.0788) (87.6953, 48.8128) (87.3048, 48.8128) knots 0 0 0 1 2 3 3 3
  line L469 (87.3048, 48.8128) -> (87.0247, 48.8128)
  line L470 (87.0247, 48.8128) -> (87.0247, 47.8311)
  line L471 (87.0247, 47.8311) -> (86.1052, 47.8311)
  line L472 (86.1052, 47.8311) -> (86.1052, 50.8811)
  line L473 (86.1052, 50.8811) -> (87.3586, 50.8811)
  spline S443 degree 2 poles (87.3586, 50.8811) (88.0037, 50.8811) (88.6007, 50.3916) (88.6007, 49.8766) knots 0 0 0 1 2 2 2
  spline S444 degree 2 poles (87.6274, 49.8427) (87.6274, 50.0294) (87.4095, 50.2218) (87.2002, 50.2218) knots 0 0 0 1 2 2 2
  line L474 (87.2002, 50.2218) -> (87.0247, 50.2218)
  line L475 (87.0247, 50.2218) -> (87.0247, 49.4692)
  line L476 (87.0247, 49.4692) -> (87.2313, 49.4692)
  spline S445 degree 2 poles (87.2313, 49.4692) (87.6274, 49.4692) (87.6274, 49.8427) knots 0 0 0 1 1 1
  line L477 (90.0889, 47.8311) -> (90.0889, 48.1621)
  line L478 (90.0889, 48.1621) -> (90.0804, 48.1621)
  spline S446 degree 2 poles (90.0804, 48.1621) (89.8625, 47.7773) (89.4155, 47.7773) knots 0 0 0 1 1 1
  spline S447 degree 2 poles (89.4155, 47.7773) (89.1071, 47.7773) (88.7591, 48.1423) (88.7591, 48.4507) knots 0 0 0 1 2 2 2
  spline S448 degree 2 poles (88.7591, 48.4507) (88.7591, 49.0929) (89.5485, 49.1948) knots 0 0 0 1 1 1
  line L479 (89.5485, 49.1948) -> (90.0889, 49.2655)
  spline S449 degree 2 poles (90.0889, 49.2655) (90.0889, 49.373) (89.8965, 49.5088) (89.7352, 49.5088) knots 0 0 0 1 2 2 2
  spline S450 degree 2 poles (89.7352, 49.5088) (89.3702, 49.5088) (88.9628, 49.2995) knots 0 0 0 1 1 1
  line L480 (88.9628, 49.2995) -> (88.9628, 49.888)
  spline S451 degree 2 poles (88.9628, 49.888) (89.1382, 49.9644) (89.673, 50.0634) (89.8625, 50.0634) knots 0 0 0 1 2 2 2
  spline S452 degree 2 poles (89.8625, 50.0634) (90.4171, 50.0634) (90.9179, 49.5881) (90.9179, 49.0335) knots 0 0 0 1 2 2 2
  line L481 (90.9179, 49.0335) -> (90.9179, 47.8311)
  line L482 (90.9179, 47.8311) -> (90.0889, 47.8311)
  spline S453 degree 2 poles (89.5513, 48.5723) (89.5513, 48.4846) (89.6645, 48.3686) (89.7692, 48.3686) knots 0 0 0 1 2 2 2
  spline S454 degree 2 poles (89.7692, 48.3686) (89.9106, 48.3686) (90.0889, 48.5808) (90.0889, 48.7478) knots 0 0 0 1 2 2 2
  line L483 (90.0889, 48.7478) -> (90.0889, 48.8298)
  line L484 (90.0889, 48.8298) -> (89.7805, 48.7874)
  spline S455 degree 2 poles (89.7805, 48.7874) (89.5513, 48.7478) (89.5513, 48.5723) knots 0 0 0 1 1 1
  spline S456 degree 2 poles (93.7811, 48.9854) (93.7811, 48.6289) (93.5378, 48.08) (93.0965, 47.7773) (92.8192, 47.7773) knots 0 0 0 1 2 3 3 3
  spline S457 degree 2 poles (92.8192, 47.7773) (92.4372, 47.7773) (92.2392, 48.0574) knots 0 0 0 1 1 1
  line L485 (92.2392, 48.0574) -> (92.2307, 48.0574)
  line L486 (92.2307, 48.0574) -> (92.2307, 46.8295)
  line L487 (92.2307, 46.8295) -> (91.3253, 46.8295)
  line L488 (91.3253, 46.8295) -> (91.3253, 50.0096)
  line L489 (91.3253, 50.0096) -> (92.2307, 50.0096)
  line L490 (92.2307, 50.0096) -> (92.2307, 49.7125)
  line L491 (92.2307, 49.7125) -> (92.2392, 49.7125)
  spline S458 degree 2 poles (92.2392, 49.7125) (92.3467, 49.8766) (92.6919, 50.0634) (92.9125, 50.0634) knots 0 0 0 1 2 2 2
  spline S459 degree 2 poles (92.9125, 50.0634) (93.3313, 50.0634) (93.7811, 49.5004) (93.7811, 48.9854) knots 0 0 0 1 2 2 2
  spline S460 degree 2 poles (92.8616, 48.96) (92.8616, 49.1637) (92.7032, 49.3985) (92.5362, 49.3985) knots 0 0 0 1 2 2 2
  spline S461 degree 2 poles (92.5362, 49.3985) (92.392, 49.3985) (92.2137, 49.1523) (92.2137, 48.9373) knots 0 0 0 1 2 2 2
  line L492 (92.2137, 48.9373) -> (92.2137, 48.8949)
  spline S462 degree 2 poles (92.2137, 48.8949) (92.2137, 48.6883) (92.3665, 48.4422) (92.5193, 48.4422) knots 0 0 0 1 2 2 2
  spline S463 degree 2 poles (92.5193, 48.4422) (92.6834, 48.4422) (92.8616, 48.711) (92.8616, 48.96) knots 0 0 0 1 2 2 2
  line L493 (95.3316, 47.8311) -> (95.3316, 48.1621)
  line L494 (95.3316, 48.1621) -> (95.3231, 48.1621)
  spline S464 degree 2 poles (95.3231, 48.1621) (95.1053, 47.7773) (94.6582, 47.7773) knots 0 0 0 1 1 1
  spline S465 degree 2 poles (94.6582, 47.7773) (94.3498, 47.7773) (94.0018, 48.1423) (94.0018, 48.4507) knots 0 0 0 1 2 2 2
  spline S466 degree 2 poles (94.0018, 48.4507) (94.0018, 49.0929) (94.7912, 49.1948) knots 0 0 0 1 1 1
  line L495 (94.7912, 49.1948) -> (95.3316, 49.2655)
  spline S467 degree 2 poles (95.3316, 49.2655) (95.3316, 49.373) (95.1392, 49.5088) (94.9779, 49.5088) knots 0 0 0 1 2 2 2
  spline S468 degree 2 poles (94.9779, 49.5088) (94.613, 49.5088) (94.2055, 49.2995) knots 0 0 0 1 1 1
  line L496 (94.2055, 49.2995) -> (94.2055, 49.888)
  spline S469 degree 2 poles (94.2055, 49.888) (94.381, 49.9644) (94.9157, 50.0634) (95.1053, 50.0634) knots 0 0 0 1 2 2 2
  spline S470 degree 2 poles (95.1053, 50.0634) (95.6598, 50.0634) (96.1606, 49.5881) (96.1606, 49.0335) knots 0 0 0 1 2 2 2
  line L497 (96.1606, 49.0335) -> (96.1606, 47.8311)
  line L498 (96.1606, 47.8311) -> (95.3316, 47.8311)
  line L499 (94.9723, 50.3548) -> (94.214, 51.0367)
  line L500 (94.214, 51.0367) -> (94.9751, 51.0367)
  line L501 (94.9751, 51.0367) -> (95.6117, 50.3548)
  line L502 (95.6117, 50.3548) -> (94.9723, 50.3548)
  spline S471 degree 2 poles (94.794, 48.5723) (94.794, 48.4846) (94.9072, 48.3686) (95.0119, 48.3686) knots 0 0 0 1 2 2 2
  spline S472 degree 2 poles (95.0119, 48.3686) (95.1534, 48.3686) (95.3316, 48.5808) (95.3316, 48.7478) knots 0 0 0 1 2 2 2
  line L503 (95.3316, 48.7478) -> (95.3316, 48.8298)
  line L504 (95.3316, 48.8298) -> (95.0232, 48.7874)
  spline S473 degree 2 poles (95.0232, 48.7874) (94.794, 48.7478) (94.794, 48.5723) knots 0 0 0 1 1 1
  line L505 (99.9915, 47.8311) -> (98.9164, 49.3023)
  spline S474 degree 2 poles (98.9164, 49.3023) (98.789, 49.4749) (98.707, 49.6164) knots 0 0 0 1 1 1
  line L506 (98.707, 49.6164) -> (98.6985, 49.6164)
  spline S475 degree 2 poles (98.6985, 49.6164) (98.7126, 49.39) (98.7126, 49.1099) knots 0 0 0 1 1 1
  line L507 (98.7126, 49.1099) -> (98.7126, 47.8311)
  line L508 (98.7126, 47.8311) -> (97.861, 47.8311)
  line L509 (97.861, 47.8311) -> (97.861, 50.8811)
  line L510 (97.861, 50.8811) -> (98.7296, 50.8811)
  line L511 (98.7296, 50.8811) -> (99.7595, 49.4805)
  spline S476 degree 2 poles (99.7595, 49.4805) (99.7793, 49.4523) (99.8359, 49.3759) (99.8896, 49.2966) (99.9377, 49.2202) (99.9519, 49.1891) knots 0 0 0 1 2 3 4 4 4
  line L512 (99.9519, 49.1891) -> (99.9604, 49.1891)
  spline S477 degree 2 poles (99.9604, 49.1891) (99.9462, 49.2825) (99.9462, 49.5117) knots 0 0 0 1 1 1
  line L513 (99.9462, 49.5117) -> (99.9462, 50.8811)
  line L514 (99.9462, 50.8811) -> (100.7978, 50.8811)
  line L515 (100.7978, 50.8811) -> (100.7978, 47.8311)
  line L516 (100.7978, 47.8311) -> (99.9915, 47.8311)
  line L517 (101.3156, 47.8311) -> (101.3156, 50.0096)
  line L518 (101.3156, 50.0096) -> (102.221, 50.0096)
  line L519 (102.221, 50.0096) -> (102.221, 47.8311)
  line L520 (102.221, 47.8311) -> (101.3156, 47.8311)
  spline S478 degree 2 poles (102.2747, 50.5981) (102.2747, 50.4057) (101.9946, 50.1681) (101.7683, 50.1681) knots 0 0 0 1 2 2 2
  spline S479 degree 2 poles (101.7683, 50.1681) (101.5476, 50.1681) (101.2647, 50.4142) (101.2647, 50.5981) knots 0 0 0 1 2 2 2
  spline S480 degree 2 poles (101.2647, 50.5981) (101.2647, 50.7849) (101.5391, 51.0169) (101.7683, 51.0169) knots 0 0 0 1 2 2 2
  spline S481 degree 2 poles (101.7683, 51.0169) (101.9946, 51.0169) (102.2747, 50.7849) (102.2747, 50.5981) knots 0 0 0 1 2 2 2
  spline S482 degree 2 poles (104.4505, 47.8933) (104.3628, 47.8424) (103.9893, 47.7773) (103.746, 47.7773) knots 0 0 0 1 2 2 2
  spline S483 degree 2 poles (103.746, 47.7773) (103.4008, 47.7773) (102.8576, 48.0574) (102.5605, 48.5582) (102.5605, 48.8722) knots 0 0 0 1 2 3 3 3
  spline S484 degree 2 poles (102.5605, 48.8722) (102.5605, 49.2457) (102.8774, 49.7805) (103.4631, 50.0634) (103.8507, 50.0634) knots 0 0 0 1 2 3 3 3
  spline S485 degree 2 poles (103.8507, 50.0634) (104.0629, 50.0634) (104.4024, 50.0068) (104.4505, 49.9728) knots 0 0 0 1 2 2 2
  line L521 (104.4505, 49.9728) -> (104.4505, 49.2655)
  spline S486 degree 2 poles (104.4505, 49.2655) (104.3826, 49.3193) (104.1279, 49.3985) (104.0204, 49.3985) knots 0 0 0 1 2 2 2
  spline S487 degree 2 poles (104.0204, 49.3985) (103.7545, 49.3985) (103.48, 49.1467) (103.48, 48.9175) knots 0 0 0 1 2 2 2
  spline S488 degree 2 poles (103.48, 48.9175) (103.48, 48.6912) (103.7488, 48.4422) (103.9865, 48.4422) knots 0 0 0 1 2 2 2
  spline S489 degree 2 poles (103.9865, 48.4422) (104.2383, 48.4422) (104.4505, 48.561) knots 0 0 0 1 1 1
  line L522 (104.4505, 48.561) -> (104.4505, 47.8933)
  spline S490 degree 2 poles (107.2345, 48.96) (107.2345, 48.4082) (106.5696, 47.7773) (105.9727, 47.7773) knots 0 0 0 1 2 2 2
  spline S491 degree 2 poles (105.9727, 47.7773) (105.3785, 47.7773) (104.7164, 48.3913) (104.7164, 48.9345) knots 0 0 0 1 2 2 2
  spline S492 degree 2 poles (104.7164, 48.9345) (104.7164, 49.2797) (105.0277, 49.7918) (105.602, 50.0634) (105.9755, 50.0634) knots 0 0 0 1 2 3 3 3
  spline S493 degree 2 poles (105.9755, 50.0634) (106.3631, 50.0634) (106.9318, 49.7776) (107.2345, 49.2712) (107.2345, 48.96) knots 0 0 0 1 2 3 3 3
  spline S494 degree 2 poles (106.315, 48.9543) (106.315, 49.3985) (105.9755, 49.3985) knots 0 0 0 1 1 1
  spline S495 degree 2 poles (105.9755, 49.3985) (105.636, 49.3985) (105.636, 48.9345) knots 0 0 0 1 1 1
  spline S496 degree 2 poles (105.636, 48.9345) (105.636, 48.4422) (105.9811, 48.4422) knots 0 0 0 1 1 1
  spline S497 degree 2 poles (105.9811, 48.4422) (106.315, 48.4422) (106.315, 48.9543) knots 0 0 0 1 1 1
  line L523 (107.5741, 47.8311) -> (107.5741, 51.0565)
  line L524 (107.5741, 51.0565) -> (108.4794, 51.0565)
  line L525 (108.4794, 51.0565) -> (108.4794, 47.8311)
  line L526 (108.4794, 47.8311) -> (107.5741, 47.8311)
  spline S498 degree 2 poles (111.337, 48.96) (111.337, 48.4082) (110.6721, 47.7773) (110.0752, 47.7773) knots 0 0 0 1 2 2 2
  spline S499 degree 2 poles (110.0752, 47.7773) (109.481, 47.7773) (108.8189, 48.3913) (108.8189, 48.9345) knots 0 0 0 1 2 2 2
  spline S500 degree 2 poles (108.8189, 48.9345) (108.8189, 49.2797) (109.1302, 49.7918) (109.7045, 50.0634) (110.078, 50.0634) knots 0 0 0 1 2 3 3 3
  spline S501 degree 2 poles (110.078, 50.0634) (110.4656, 50.0634) (111.0343, 49.7776) (111.337, 49.2712) (111.337, 48.96) knots 0 0 0 1 2 3 3 3
  spline S502 degree 2 poles (110.4175, 48.9543) (110.4175, 49.3985) (110.078, 49.3985) knots 0 0 0 1 1 1
  spline S503 degree 2 poles (110.078, 49.3985) (109.7385, 49.3985) (109.7385, 48.9345) knots 0 0 0 1 1 1
  spline S504 degree 2 poles (109.7385, 48.9345) (109.7385, 48.4422) (110.0837, 48.4422) knots 0 0 0 1 1 1
  spline S505 degree 2 poles (110.0837, 48.4422) (110.4175, 48.4422) (110.4175, 48.9543) knots 0 0 0 1 1 1
  line L527 (109.9705, 50.3548) -> (109.2122, 51.0367)
  line L528 (109.2122, 51.0367) -> (109.9733, 51.0367)
  line L529 (109.9733, 51.0367) -> (110.6099, 50.3548)
  line L530 (110.6099, 50.3548) -> (109.9705, 50.3548)
  spline S506 degree 2 poles (69.93, 42.9327) (69.93, 42.7686) (69.7603, 42.4772) (69.4689, 42.3103) (69.3076, 42.3103) knots 0 0 0 1 2 3 3 3
  spline S507 degree 2 poles (69.3076, 42.3103) (69.0558, 42.3103) (68.6936, 42.6725) (68.6936, 42.9327) knots 0 0 0 1 2 2 2
  spline S508 degree 2 poles (68.6936, 42.9327) (68.6936, 43.1846) (69.0501, 43.5467) (69.3076, 43.5467) knots 0 0 0 1 2 2 2
  spline S509 degree 2 poles (69.3076, 43.5467) (69.5707, 43.5467) (69.93, 43.1789) (69.93, 42.9327) knots 0 0 0 1 2 2 2
  spline S510 degree 2 poles (80.6843, 43.459) (80.6843, 42.995) (80.2938, 42.282) (79.5723, 41.8944) (79.0998, 41.8944) knots 0 0 0 1 2 3 3 3
  line L531 (79.0998, 41.8944) -> (77.8068, 41.8944)
  line L532 (77.8068, 41.8944) -> (77.8068, 44.9444)
  line L533 (77.8068, 44.9444) -> (79.0715, 44.9444)
  spline S511 degree 2 poles (79.0715, 44.9444) (80.6843, 44.9444) (80.6843, 43.459) knots 0 0 0 1 1 1
  spline S512 degree 2 poles (79.7081, 43.4505) (79.7081, 43.6712) (79.5271, 44.0305) (79.1904, 44.2257) (78.964, 44.2257) knots 0 0 0 1 2 3 3 3
  line L534 (78.964, 44.2257) -> (78.7264, 44.2257)
  line L535 (78.7264, 44.2257) -> (78.7264, 42.613)
  line L536 (78.7264, 42.613) -> (78.9838, 42.613)
  spline S513 degree 2 poles (78.9838, 42.613) (79.3149, 42.613) (79.7081, 43.0657) (79.7081, 43.4505) knots 0 0 0 1 2 2 2
  line L537 (81.0323, 41.8944) -> (81.0323, 44.073)
  line L538 (81.0323, 44.073) -> (81.9376, 44.073)
  line L539 (81.9376, 44.073) -> (81.9376, 41.8944)
  line L540 (81.9376, 41.8944) -> (81.0323, 41.8944)
  spline S514 degree 2 poles (81.9914, 44.6615) (81.9914, 44.4691) (81.7113, 44.2314) (81.485, 44.2314) knots 0 0 0 1 2 2 2
  spline S515 degree 2 poles (81.485, 44.2314) (81.2643, 44.2314) (80.9813, 44.4776) (80.9813, 44.6615) knots 0 0 0 1 2 2 2
  spline S516 degree 2 poles (80.9813, 44.6615) (80.9813, 44.8482) (81.2558, 45.0802) (81.485, 45.0802) knots 0 0 0 1 2 2 2
  spline S517 degree 2 poles (81.485, 45.0802) (81.7113, 45.0802) (81.9914, 44.8482) (81.9914, 44.6615) knots 0 0 0 1 2 2 2
  line L541 (85.4064, 41.8944) -> (84.3737, 41.8944)
  line L542 (84.3737, 41.8944) -> (83.3891, 44.9444)
  line L543 (83.3891, 44.9444) -> (84.3765, 44.9444)
  line L544 (84.3765, 44.9444) -> (84.8433, 43.0657)
  spline S518 degree 2 poles (84.8433, 43.0657) (84.8999, 42.8394) (84.9056, 42.7262) knots 0 0 0 1 1 1
  line L545 (84.9056, 42.7262) -> (84.9254, 42.7262)
  spline S519 degree 2 poles (84.9254, 42.7262) (84.9395, 42.8677) (84.9933, 43.0799) knots 0 0 0 1 1 1
  line L546 (84.9933, 43.0799) -> (85.446, 44.9444)
  line L547 (85.446, 44.9444) -> (86.4023, 44.9444)
  line L548 (86.4023, 44.9444) -> (85.4064, 41.8944)
  line L549 (86.6428, 41.8944) -> (86.6428, 44.073)
  line L550 (86.6428, 44.073) -> (87.5482, 44.073)
  line L551 (87.5482, 44.073) -> (87.5482, 41.8944)
  line L552 (87.5482, 41.8944) -> (86.6428, 41.8944)
  spline S520 degree 2 poles (87.6019, 44.6615) (87.6019, 44.4691) (87.3218, 44.2314) (87.0955, 44.2314) knots 0 0 0 1 2 2 2
  spline S521 degree 2 poles (87.0955, 44.2314) (86.8748, 44.2314) (86.5919, 44.4776) (86.5919, 44.6615) knots 0 0 0 1 2 2 2
  spline S522 degree 2 poles (86.5919, 44.6615) (86.5919, 44.8482) (86.8663, 45.0802) (87.0955, 45.0802) knots 0 0 0 1 2 2 2
  spline S523 degree 2 poles (87.0955, 45.0802) (87.3218, 45.0802) (87.6019, 44.8482) (87.6019, 44.6615) knots 0 0 0 1 2 2 2
  line L553 (89.3957, 41.8944) -> (89.3957, 43.0827)
  spline S524 degree 2 poles (89.3957, 43.0827) (89.3957, 43.2864) (89.2741, 43.4618) (89.1382, 43.4618) knots 0 0 0 1 2 2 2
  spline S525 degree 2 poles (89.1382, 43.4618) (89.0222, 43.4618) (88.8893, 43.2779) (88.8893, 43.1365) knots 0 0 0 1 2 2 2
  line L554 (88.8893, 43.1365) -> (88.8893, 41.8944)
  line L555 (88.8893, 41.8944) -> (87.9839, 41.8944)
  line L556 (87.9839, 41.8944) -> (87.9839, 44.073)
  line L557 (87.9839, 44.073) -> (88.8893, 44.073)
  line L558 (88.8893, 44.073) -> (88.8893, 43.7334)
  line L559 (88.8893, 43.7334) -> (88.8978, 43.7334)
  spline S526 degree 2 poles (88.8978, 43.7334) (89.0053, 43.9202) (89.3731, 44.1267) (89.5881, 44.1267) knots 0 0 0 1 2 2 2
  spline S527 degree 2 poles (89.5881, 44.1267) (90.3011, 44.1267) (90.3011, 43.2242) knots 0 0 0 1 1 1
  line L560 (90.3011, 43.2242) -> (90.3011, 41.8944)
  line L561 (90.3011, 41.8944) -> (89.3957, 41.8944)
  spline S528 degree 2 poles (92.5051, 41.9566) (92.4174, 41.9057) (92.0439, 41.8406) (91.8006, 41.8406) knots 0 0 0 1 2 2 2
  spline S529 degree 2 poles (91.8006, 41.8406) (91.4555, 41.8406) (90.9122, 42.1207) (90.6151, 42.6215) (90.6151, 42.9356) knots 0 0 0 1 2 3 3 3
  spline S530 degree 2 poles (90.6151, 42.9356) (90.6151, 43.309) (90.932, 43.8438) (91.5177, 44.1267) (91.9053, 44.1267) knots 0 0 0 1 2 3 3 3